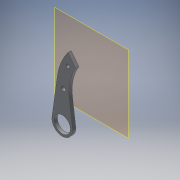
# Autodesk Inventor part: FrontMotorPlateA
Saved by Autodesk Inventor 2019.3 (Build 233278000, 278)
## iProperties
Created: 2019-05-08
Part Number: FrontMotorPlateA
Material: Generic
Document SubType Name: Modeling
Designer: eroldan
Density: 1 g/cm^3
Appearance: Default
Author: eroldan
Autodesk Inventor part; units mm, degrees
ref_plane "YZ Plane" through (0, 0, 0) normal (1, 0, 0) x (0, 1, 0)
ref_plane "XZ Plane" through (0, 0, 0) normal (0, 1, 0) x (-1, 0, 0)
ref_plane "XY Plane" through (0, 0, 0) normal (0, 0, 1) x (1, 0, 0)
ref_plane "Work Plane1" through (0, 0, 0) normal (0, 0, 1) x (1, 0, 0)
sketch "Sketch1" plane through (0, 0, 0) normal (0, 0, 1) x (1, 0, 0)
  circle A0 centre (-29.429, -82.1546) radius 11.1125 projected
  circle A1 centre (-27.8641, -39.0242) radius 3 projected
  arc A2 (-43.404, -80.1898) -> (-15.4377, -80.3088) centre (-29.429, -82.1546) ccw projected
  line L0 (-19.8487, -46.8714) -> (-15.4377, -80.3088) projected
  line L1 (-43.404, -80.1898) -> (-36.1191, -28.3736) projected
  line L2 (-10.9618, -6.7771) -> (-21.6846, 6.7146) projected
  arc A3 (-10.9618, -6.7771) -> (-19.8487, -46.8714) centre (39.6359, -39.0242) ccw
  arc A4 (-21.6846, 6.7146) -> (-36.1191, -28.3736) centre (39.6359, -39.0242) ccw
  circle A5 centre (-21.8255, -9.1802) radius 2.5 projected
  point P0 (0, 0)
  point P1 (69.9962, 12.7276)
  point P2 (71.0345, 12.3011)
  constraints: 4 point on circle, 2 centre point, 2 end point
extrude "Extrusion1" add sketch "Sketch1" along normal blind 4.4
body "Solid1"
